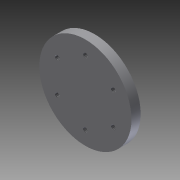
# Autodesk Inventor part: wheel hub
Saved by Autodesk Inventor 2012 (Build 160160000, 160)
## iProperties
Created: 2011-12-01
Part Number: wheel hub
Material: Default
Document SubType Name: Modeling
Designer: Antonella
Density: 1 g/cm^3
Author: Antonella
Autodesk Inventor part; units mm, degrees
ref_plane "YZ Plane" through (0, 0, 0) normal (1, 0, 0) x (0, 1, 0)
ref_plane "XZ Plane" through (0, 0, 0) normal (0, 1, 0) x (-1, 0, 0)
ref_plane "XY Plane" through (0, 0, 0) normal (0, 0, 1) x (1, 0, 0)
sketch "Sketch1" plane through (0, 0, 0) normal (0, 0, 1) x (1, 0, 0)
  line L0 (-142.24, 0) -> (142.24, 0) projected
  line L1 (0, -142.24) -> (0, 142.24) projected
  circle A0 centre (0, 0) radius 63.5
  circle A1 centre (0, 0) radius 50.8 construction
  circle A2 centre (0, 0) radius 101.6 construction
  dimension "d0" = 101.6
  dimension "d1" = 127
  dimension "d20" = 203.2
  constraints: 3 centre point, 3 coincident
  measures "d0" diameter of A1
  measures "d1" diameter of A0
  measures "d20" diameter of A2
extrude "Extrusion1" add sketch "Sketch1" along normal blind 12.7
sketch "Sketch4" plane through (0, 0, 12.7) normal (0, 0, 1) x (1, 0, 0)
  line L0 (-88.9, 0) -> (88.9, 0) projected
  line L1 (0, -88.9) -> (0, 88.9) projected
  point P0 (0, 44.45)
  dimension "d21" = 44.45
  measures "d21" distance from line of L0 point (0, 44.45)
hole "Hole2" at (0, 44.45, 12.7) direction (0, 0, -1) diameter 6.4008 end through all thread size "5/16-18 UNC" class "2B" standard "ANSI Unified Screw Threads"
pattern_circular "Circular Pattern1" count 6 over 360 about axis through (0, 0, -10) along (0, 0, 1) of "Hole2"
body "Solid1"
